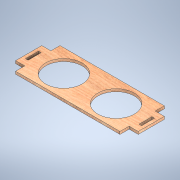
# Autodesk Inventor part: Parte C
Saved by Autodesk Inventor 2022 (Build 260153000, 153)
## iProperties
Created: 2023-02-12
Part Number: Parte C
Material: Madera (abedul)
Document SubType Name: Modeling
Designer: USUARIO
Density: 0.55 g/cm^3
Appearance: Abedul - Natural pulido
Author: USUARIO
Autodesk Inventor part; units mm, degrees
ref_plane "YZ Plane" through (0, 0, 0) normal (1, 0, 0) x (0, 1, 0)
ref_plane "XZ Plane" through (0, 0, 0) normal (0, 1, 0) x (-1, 0, 0)
ref_plane "XY Plane" through (0, 0, 0) normal (0, 0, 1) x (1, 0, 0)
sketch "Boceto1" plane through (0, 0, 0) normal (0, 1, 0) x (-1, 0, 0)
  line L0 (200, 85) -> (-200, 85)
  line L1 (-200, 85) -> (-200, -85)
  line L2 (-200, -85) -> (200, -85)
  line L3 (200, -85) -> (200, 85)
  line L4 (200, 85) -> (-200, -85) construction
  line L5 (-200, 85) -> (200, -85) construction
  point P0 (0, 0)
  dimension "d0" = 400
  dimension "d1" = 170
  constraints: 12 end point, 2 midpoint, 2 parallel, 1 horizontal, 1 perpendicular
  measures "d0" distance of L2.end L1.end
  measures "d1" distance of L1.end L0.end
extrude "Extrusión1" add sketch "Boceto1" along normal blind 10
sketch "Boceto2" plane through (0, 10, 0) normal (0, 1, 0) x (1, 0, 0)
  line L0 (0, 0) -> (-100, 0)
  line L1 (0, 0) -> (100, 0) construction
  circle A0 centre (-100, 0) radius 70
  line L2 (0, 0) -> (0, 85)
  line L3 (200, 85) -> (-200, 85) projected
  circle A1 centre (100, 0) radius 70
  dimension "d5" = 100
  dimension "d6" = 180
  dimension "d7" = 140
  constraints: 6 end point, 2 centre point, 2 horizontal, 1 coincident, 1 collinear, 1 midpoint, 1 symmetric about line, 1 other
  measures "d5" distance of L0.start L0.end
  measures "d6" angle of L0 L1
  measures "d7" diameter of A0
extrude "Extrusión2" cut sketch "Boceto2" against normal up to surface (10 mm away)
sketch "Boceto3" plane through (0, 10, 0) normal (0, 1, 0) x (1, 0, 0)
  line L0 (165, 50) -> (235, 50)
  line L1 (235, 50) -> (235, -50)
  line L2 (235, -50) -> (165, -50)
  line L3 (165, -50) -> (165, 50)
  line L4 (200, -85) -> (200, 85) projected
  line L5 (165, 50) -> (235, -50) construction
  line L6 (235, 50) -> (165, -50) construction
  line L7 (200, 50) -> (200, -50)
  line L8 (0, -85) -> (0, 85)
  line L9 (200, 85) -> (-200, 85) projected
  line L10 (-165, 50) -> (-235, 50)
  line L11 (-235, 50) -> (-235, -50)
  line L12 (-235, -50) -> (-165, -50)
  line L13 (-200, -85) -> (-200, 85)
  point P0 (0, 0)
  point P1 (200, 0)
  point P2 (-200, -50)
  point P3 (-200, 50)
  dimension "d10" = 70
  dimension "d11" = 100
  constraints: 24 end point, 6 midpoint, 5 symmetric about line, 2 parallel, 2 point on line, 1 horizontal, 1 perpendicular
  measures "d10" distance of L1.end L2.end
  measures "d11" distance of L0.end L1.end
extrude "Extrusión3" add sketch "Boceto3" against normal up to surface (10 mm away) contours L0 L1 L2 L4 | L13 L12 L11 L10
sketch "Boceto4" plane through (0, 10, 0) normal (0, 1, 0) x (1, 0, 0)
  line L0 (0, 0) -> (0, 85)
  line L1 (200, 85) -> (-200, 85) projected
  line L2 (-235, 50) -> (-235, -50) projected
  line L3 (-235, 0) -> (-217.5, 0)
  line L4 (-235, 0) -> (-217.5, 0) construction
  line L5 (-222.5, -25) -> (-212.5, -25)
  line L6 (-212.5, -25) -> (-212.5, 25)
  line L7 (-212.5, 25) -> (-222.5, 25)
  line L8 (-222.5, 25) -> (-222.5, -25)
  line L9 (-222.5, -25) -> (-212.5, 25) construction
  line L10 (-212.5, -25) -> (-222.5, 25) construction
  line L11 (222.5, -25) -> (212.5, -25)
  line L12 (212.5, -25) -> (212.5, 25)
  line L13 (212.5, 25) -> (222.5, 25)
  line L14 (222.5, 25) -> (222.5, -25)
  dimension "d14" = 17.5
  dimension "d15" = 0
  dimension "d16" = 10
  dimension "d17" = 50
  constraints: 26 end point, 4 midpoint, 4 symmetric about line, 3 horizontal, 2 parallel, 1 collinear, 1 perpendicular
  measures "d14" distance of L3.start L3.end
  measures "d15" distance between parallel lines of L3 L4
  measures "d16" distance of L7.end L6.end
  measures "d17" distance of L6.end L5.end
extrude "Extrusión4" cut sketch "Boceto4" against normal up to surface (10 mm away)
equation "\"d0\" = largo_c"
equation "\"d1\" = ancho_c"
equation "\"d2\" = grueso"
equation "\"d5\" = d_plato"
equation "\"d7\" = diametro_c"
equation "\"d10\" = largo_p"
equation "\"d11\" = ancho_p"
equation "\"d14\" = 0.25 * largo_p"
equation "\"d16\" = ancho_a"
equation "\"d17\" = alto_a"
equation "\"ancho_c\" = 170"
equation "\"largo_c\" = 400"
equation "\"grueso\" = 10"
equation "\"diametro_c\" = 140"
equation "\"d_plato\" = 100"
equation "\"ancho_p\" = 100"
equation "\"largo_p\" = 70"
equation "\"ancho_a\" = 10"
equation "\"alto_a\" = 50"
